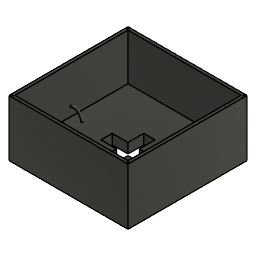
body (Autodesk Fusion 360 design; units mm, degrees)
part number: 2026-06-04-19-50-26-634
Autodesk Fusion 360 part; units mm, degrees
sketch "Sketch1" plane through (0, 0, 0) normal (0, 0, 1) x (1, 0, 0)
  line L0 (0, 0) -> (560, 0)
  line L1 (560, 0) -> (560, -560)
  line L2 (560, -560) -> (0, -560)
  line L3 (0, -560) -> (0, 0)
  line L4 (253.6071, -253.6071) -> (306.3929, -306.3929) construction
  line L5 (306.3929, -253.6071) -> (253.6071, -306.3929) construction
  line L6 (0, 0) -> (560, -560) construction
  line L7 (560, 0) -> (0, -560) construction
  line L8 (308, -252) -> (308, -174)
  line L9 (308, -174) -> (252, -174)
  line L10 (252, -174) -> (252, -252)
  line L11 (308, -308) -> (308, -386)
  line L12 (308, -386) -> (252, -386)
  line L13 (252, -386) -> (252, -308)
  line L14 (252, -252) -> (174, -252)
  line L15 (174, -252) -> (174, -308)
  line L16 (174, -308) -> (252, -308)
  line L17 (308, -252) -> (386, -252)
  line L18 (386, -252) -> (386, -308)
  line L19 (386, -308) -> (308, -308)
  point P0 (280, -280)
  point P1 (280, -280)
  point P2 (308, -308)
  point P3 (308, -308)
  point P4 (310, -304.226)
  point P5 (249.7112, -304.226)
  point P6 (252, -308)
  point P7 (252, -308)
  point P8 (252, -252)
  point P9 (252, -252)
  point P10 (249.7112, -243.9373)
  point P11 (310, -243.9373)
  point P12 (308, -252)
  point P13 (308, -252)
  dimension "d1" = 560
  dimension "d39" = 56
  dimension "d40" = 56
  dimension "d41" = 78
  constraint horizontal L0
  constraint vertical L1
  constraint horizontal L2
  constraint vertical L3
  constraint equal L0 L3
  constraint coincident L0.start L3.end
  constraint midpoint L5 P1
  constraint midpoint L7 P1
  constraint coincident P1 P0
  constraint vertical L8
  constraint horizontal L9
  constraint vertical L10
  constraint vertical L11
  constraint horizontal L12
  constraint vertical L13
  constraint horizontal L14
  constraint vertical L15
  constraint horizontal L16
  constraint horizontal L17
  constraint vertical L18
  constraint horizontal L19
  constraint equal L16 L19
  constraint equal L8 L17
  constraint equal L11 L19
  constraint equal L15 L18
  constraint equal L9 L15
  constraint equal L9 L12
  constraint collinear L16 L19
  constraint collinear L8 L11
  constraint coincident P3 P2
  constraint coincident P7 P6
  constraint coincident P9 P8
  constraint coincident P13 L8.start
  constraint coincident P13 P12
  constraint coincident L6 P3
  constraint coincident L7 P13
  constraint coincident L6 P9
  measures "d1" distance of L0.start L0.end
  measures "d39" distance of L8 L10
  measures "d40" distance of L14 L16
  measures "d41" distance of L8.start L8.end
extrude "Extrude1" add sketch "Sketch1" along normal blind 280 thin wall 15 on the left open curves L3 L0 L1 L2
extrude "Extrude2" add sketch "Sketch1" along normal blind 50
sketch "Sketch2" plane through (0, 0, 0) normal (0, -1, 0) x (1, 0, 0)
  line L0 (0, 50) -> (560, 50)
  line L1 (560, 50) -> (560, 280)
  line L2 (560, 280) -> (0, 280)
  line L3 (0, 280) -> (0, 50)
  spline S0 degree 5 poles (560, 94.8263, 0) (557.9932, 95.2995, 1.2647) (554.0734, 96.1248, 3.6823) (548.4758, 96.9994, 6.9732) (541.5853, 97.4267, 10.6789) (533.9913, 96.6472, 14.0981) (527.5032, 94.4421, 16.201) (522.205, 90.7031, 16.8876) (518.1308, 85.3863, 16.1174) (515.2192, 78.5709, 13.9635) (513.3768, 70.3771, 10.5368) (512.6854, 62.8133, 6.8642) (512.5786, 56.6097, 3.6196) (512.6875, 52.2419, 1.2422) (512.7869, 50, 0) knots 0 0 0 0 0 0 0.1 0.2 0.3 0.4 0.5 0.6 0.7 0.8 0.9 1 1 1 1 1 1
  point P0 (523.1531, 90.9057)
ref_plane "WorkPlane1" through (0, -275, 0) normal (0, 1, 0) x (0, 0, 1)
ref_plane "WorkPlane2" through (0, -275, 0) normal (0, -1, 0) x (1, 0, 0)
sketch "Sketch3" plane through (0, -275, 0) normal (0, -1, 0) x (-1, 0, 0)
  spline S0 degree 5 poles (-559.2194, -95.4249, 1.7664) (-557.1869, -96.2217, 1.8575) (-553.2228, -97.6631, 2.0373) (-547.5796, -99.3689, 2.3) (-540.6712, -100.7159, 2.6356) (-533.129, -100.753, 3.0295) (-526.7673, -99.0122, 3.3955) (-521.6658, -95.3735, 3.7318) (-517.8375, -89.8175, 4.0381) (-515.2023, -82.4645, 4.3163) (-513.6567, -73.4704, 4.5689) (-513.2142, -65.0794, 4.7522) (-513.2995, -58.1579, 4.8799) (-513.5388, -53.2689, 4.9607) (-513.704, -50.7558, 5) knots 0 0 0 0 0 0 0.1 0.2 0.3 0.4 0.5 0.6 0.7 0.8 0.9 1 1 1 1 1 1
  spline S1 degree 5 poles (2.4057, -94.8675, 7.7694) (0.51, -95.3847, 7.7637) (-3.2053, -96.2866, 7.7427) (-8.5495, -97.2416, 7.6823) (-15.2103, -97.7061, 7.5427) (-22.7116, -96.8513, 7.2638) (-29.3235, -94.449, 6.8722) (-34.988, -90.3982, 6.3605) (-39.7, -84.6897, 5.7281) (-43.522, -77.4326, 4.983) (-46.5327, -68.7636, 4.135) (-48.3508, -60.8009, 3.3818) (-49.4042, -54.2892, 2.7776) (-49.9709, -49.7121, 2.3576) (-50.2203, -47.3645, 2.1433) knots 0 0 0 0 0 0 0.1 0.2 0.3 0.4 0.5 0.6 0.7 0.8 0.9 1 1 1 1 1 1
  point P0 (-523.4754, -96.2662)
  point P1 (-32.7844, -91.6615)
pipe "Pipe1" add diameter 10 path "Sketch3" along S1
pipe "Pipe2" add diameter 10 path "Sketch3" along S0
sketch "Sketch4" plane through (0, 0, 280) normal (0, 0, 1) x (-1, 0, 0)
  line L0 (0, 0) -> (-560, 0)
  line L1 (-560, 0) -> (-560, 560)
  line L2 (-560, 560) -> (0, 560)
  line L3 (0, 560) -> (0, 0)
  line L4 (15, -15) -> (15, 575)
  line L5 (15, 575) -> (-575, 575)
  line L6 (-575, 575) -> (-575, -15)
  line L7 (-575, -15) -> (15, -15)
  circle A0 centre (7, -7) radius 5
  circle A1 centre (7, 567) radius 5
  circle A2 centre (-567, 567) radius 5
  circle A3 centre (-567, -7) radius 5
  dimension "d17" = 10
  dimension "d18" = 10
  dimension "d19" = 10
  dimension "d20" = 10
  dimension "d21" = 8
  dimension "d22" = 8
  dimension "d23" = 8
  dimension "d24" = 8
  dimension "d25" = 8
  dimension "d26" = 8
  dimension "d27" = 8
  dimension "d28" = 8
  measures "d17" diameter of A0
  measures "d18" diameter of A1
  measures "d19" diameter of A2
  measures "d20" diameter of A3
  measures "d21" distance of L7 A0.centre
  measures "d22" distance of L4 A0.centre
  measures "d23" distance of L4 A1.centre
  measures "d24" distance of L5 A1.centre
  measures "d25" distance of L6 A2.centre
  measures "d26" distance of L5 A2.centre
  measures "d27" distance of L7 A3.centre
  measures "d28" distance of L6 A3.centre
extrude "Extrude3" cut sketch "Sketch4" against normal blind 10 contours A0 | A1 | A2 | A3
thread "Thread1" "ISO Metric profile 10.0 M10x1.5 M10x1.5 6H" major diameter 10.198 minor diameter 8.526 pitch 1.5 angle 60 resizes the face on face at (-11.9938, 7.2492, 273.3333)
thread "Thread2" "ISO Metric profile 10.0 M10x1.5 M10x1.5 6H" major diameter 10.198 minor diameter 8.526 pitch 1.5 angle 60 resizes the face on face at (566.3783, 2.0388, 273.3333)
thread "Thread3" "ISO Metric profile 10.0 M10x1.5 M10x1.5 6H" major diameter 10.198 minor diameter 8.526 pitch 1.5 angle 60 resizes the face on face at (566.3783, -571.9612, 273.3333)
thread "Thread4" "ISO Metric profile 10.0 M10x1.5 M10x1.5 6H" major diameter 10.198 minor diameter 8.526 pitch 1.5 angle 60 resizes the face on face at (-10.9857, -570.019, 273.3333)
scale "Scale1" factor 0.254237 about (252, -252, 50) bodies 1
